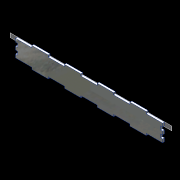
# Autodesk Inventor part: FrontArmorPlate
Saved by Autodesk Inventor 2022 (Build 260153000, 153)
## iProperties
Created: 2022-03-07
Part Number: FrontArmorPlate
Material: Aluminum 6061
Document SubType Name: Modeling
Designer: tandu
Density: 2.7 g/cm^3
Appearance: Aluminum - Flat
Thickness: 0.50000000 in
Author: tandu
Autodesk Inventor part; units mm, degrees
ref_plane "YZ Plane" through (0, 0, 0) normal (1, 0, 0) x (0, 1, 0)
ref_plane "XZ Plane" through (0, 0, 0) normal (0, 1, 0) x (-1, 0, 0)
ref_plane "Work Plane1" through (0, 0, 0) normal (0, 0, 1) x (1, 0, 0)
sketch "Sketch1" plane through (0, 0, 0) normal (0, 0, 1) x (1, 0, 0)
  line L0 (-1003.2396, -88.9) -> (-1003.2396, -63.5) projected
  line L1 (-18.9896, -88.9) -> (-1003.2396, -88.9) construction
  line L2 (-18.9896, -63.5) -> (-18.9896, -88.9) projected
  line L3 (-18.9896, -63.5) -> (-1003.2396, -63.5) construction
  line L4 (-1003.3, 0) -> (-1003.3, 25.4) projected
  line L5 (-19.05, 0) -> (-1003.3, 0) construction
  line L6 (-19.05, 25.4) -> (-19.05, 0) projected
  line L7 (-19.05, 25.4) -> (-1003.3, 25.4) construction
  line L8 (-1003.3, 25.4) -> (-18.9896, 25.4) construction
  line L9 (-18.9896, 25.4) -> (-18.9896, -88.9)
  line L10 (-18.9896, -88.9) -> (-1003.3, -88.9) construction
  line L11 (-1003.3, -88.9) -> (-1003.3, 25.4)
  line L12 (-1003.3, 25.4) -> (-990.6, 25.4)
  line L13 (-990.6, 25.4) -> (-990.6, 2.54) construction
  line L14 (-990.6, 2.54) -> (-1003.3, 2.54)
  line L15 (-1003.3, 2.54) -> (-1003.3, 25.4)
  line L16 (-1003.3, -88.9) -> (-990.6, -88.9)
  line L17 (-990.6, -88.9) -> (-990.6, -66.04) construction
  line L18 (-990.6, -66.04) -> (-1003.3, -66.04)
  line L19 (-1003.3, -66.04) -> (-1003.3, -88.9)
  line L20 (-990.6, -66.04) -> (-1003.3, -66.04)
  line L21 (-1003.3, -66.04) -> (-1003.3, -43.18)
  line L22 (-1003.3, -43.18) -> (-990.6, -43.18)
  line L23 (-990.6, -43.18) -> (-990.6, -66.04)
  line L24 (-990.6, 2.54) -> (-1003.3, 2.54)
  line L25 (-1003.3, 2.54) -> (-1003.3, -20.32)
  line L26 (-1003.3, -20.32) -> (-990.6, -20.32)
  line L27 (-990.6, -20.32) -> (-990.6, 2.54)
  line L28 (-990.6, -20.32) -> (-1003.3, -20.32)
  line L29 (-1003.3, -20.32) -> (-1003.3, -43.18)
  line L30 (-1003.3, -43.18) -> (-990.6, -43.18)
  line L31 (-990.6, -43.18) -> (-990.6, -20.32) construction
  line L32 (-511.1448, 25.4) -> (-511.1448, -88.9) construction
  line L33 (-18.9896, 0) -> (-18.9896, 25.4)
  line L34 (-18.9896, 25.4) -> (-31.6896, 25.4)
  line L35 (-31.6896, 25.4) -> (-31.6896, 2.54) construction
  line L36 (-31.6896, 2.54) -> (-18.9896, 2.54)
  line L37 (-31.6896, -88.9) -> (-31.6896, -66.04) construction
  line L38 (-31.6896, -66.04) -> (-18.9896, -66.04)
  line L39 (-18.9896, -20.32) -> (-31.6896, -20.32)
  line L40 (-18.9896, -43.18) -> (-31.6896, -43.18)
  line L41 (-31.6896, -43.18) -> (-31.6896, -20.32) construction
  line L42 (-31.6896, 2.54) -> (-31.6896, -20.32)
  line L43 (-31.6896, -43.18) -> (-31.6896, -66.04)
  line L44 (-1003.3, 25.4) -> (-893.9322, 25.4)
  line L45 (-893.9322, 25.4) -> (-893.9322, 38.1)
  line L46 (-893.9322, 38.1) -> (-1003.3, 38.1)
  line L47 (-1003.3, 38.1) -> (-1003.3, 25.4)
  line L48 (-893.9322, 38.1) -> (-784.5644, 38.1)
  line L49 (-784.5644, 38.1) -> (-784.5644, 25.4)
  line L50 (-784.5644, 25.4) -> (-893.9322, 25.4) construction
  line L51 (-893.9322, 25.4) -> (-893.9322, 38.1)
  line L52 (-784.5644, 25.4) -> (-675.1965, 25.4)
  line L53 (-675.1965, 25.4) -> (-675.1965, 38.1)
  line L54 (-675.1965, 38.1) -> (-784.5644, 38.1)
  line L55 (-784.5644, 38.1) -> (-784.5644, 25.4)
  line L56 (-675.1965, 38.1) -> (-565.8287, 38.1)
  line L57 (-565.8287, 38.1) -> (-565.8287, 25.4)
  line L58 (-565.8287, 25.4) -> (-675.1965, 25.4) construction
  line L59 (-675.1965, 25.4) -> (-675.1965, 38.1)
  line L60 (-565.8287, 38.1) -> (-456.4609, 38.1)
  line L61 (-456.4609, 38.1) -> (-456.4609, 25.4)
  line L62 (-456.4609, 25.4) -> (-565.8287, 25.4)
  line L63 (-565.8287, 25.4) -> (-565.8287, 38.1)
  line L64 (-456.4609, 38.1) -> (-347.0931, 38.1)
  line L65 (-347.0931, 38.1) -> (-347.0931, 25.4)
  line L66 (-347.0931, 25.4) -> (-456.4609, 25.4) construction
  line L67 (-456.4609, 25.4) -> (-456.4609, 38.1)
  line L68 (-347.0931, 38.1) -> (-237.7252, 38.1)
  line L69 (-237.7252, 38.1) -> (-237.7252, 25.4)
  line L70 (-237.7252, 25.4) -> (-347.0931, 25.4)
  line L71 (-347.0931, 25.4) -> (-347.0931, 38.1)
  line L72 (-237.7252, 38.1) -> (-128.3574, 38.1)
  line L73 (-128.3574, 38.1) -> (-128.3574, 25.4)
  line L74 (-128.3574, 25.4) -> (-237.7252, 25.4) construction
  line L75 (-237.7252, 25.4) -> (-237.7252, 38.1)
  line L76 (-128.3574, 38.1) -> (-18.9896, 38.1)
  line L77 (-18.9896, 38.1) -> (-18.9896, 25.4)
  line L78 (-18.9896, 25.4) -> (-128.3574, 25.4)
  line L79 (-128.3574, 25.4) -> (-128.3574, 38.1)
  line L80 (-18.9896, -31.75) -> (-1003.3, -31.75) construction
  line L81 (-893.9322, -101.6) -> (-784.5644, -101.6)
  line L82 (-784.5644, -101.6) -> (-784.5644, -88.9)
  line L83 (-893.9322, -88.9) -> (-893.9322, -101.6)
  line L84 (-675.1965, -88.9) -> (-675.1965, -101.6)
  line L85 (-675.1965, -101.6) -> (-565.8287, -101.6)
  line L86 (-456.4609, -101.6) -> (-456.4609, -88.9)
  line L87 (-565.8287, -88.9) -> (-565.8287, -101.6)
  line L88 (-456.4609, -101.6) -> (-347.0931, -101.6)
  line L89 (-347.0931, -101.6) -> (-347.0931, -88.9)
  line L90 (-237.7252, -101.6) -> (-237.7252, -88.9)
  line L91 (-237.7252, -101.6) -> (-128.3574, -101.6)
  line L92 (-128.3574, -101.6) -> (-128.3574, -88.9)
  line L93 (-990.6, -88.9) -> (-893.9322, -88.9)
  line L94 (-784.5644, -88.9) -> (-675.1965, -88.9)
  line L95 (-565.8287, -88.9) -> (-456.4609, -88.9)
  line L96 (-347.0931, -88.9) -> (-237.7252, -88.9)
  line L97 (-128.3574, -88.9) -> (-18.9896, -88.9)
  point P0 (0, 0)
  point P1 (-1003.2396, -66.04)
  point P2 (-19.05, 2.54)
  dimension "d2" = 12.7
  dimension "d3" = 12.7
  constraints: 178 end point, 29 parallel, 27 symmetric about line, 18 collinear, 15 horizontal, 14 perpendicular, 6 point on line, 3 midpoint, 2 vertical, 10 other
  measures "d2" distance between parallel lines of L4 L13
  measures "d3" distance of L46.end L4.end
extrude "Extrusion1" add sketch "Sketch1" along normal blind 12.7 contours L0 L18 L23 L22 L11 L26 L27 L14 L4 L12 L44 L45 L48 L49 L52 L53 L56 L57 L62 L61 L64 L65 L70 L69 L72 L73 L78 L34 L6 L36 L42 L39 L9 L40 L43 L38 L2 L97 L92 L91 L90 L96 L89 L88 L86 L95 L87 L85 L84 L94 L82 L81 L83 L93 L16
equation "\"d2\" = Thickness"
equation "\"d4\" = Thickness"
equation "\"Thickness\" = 12.7"
body "Solid1"
